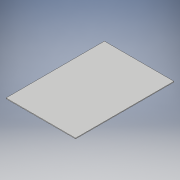
# Autodesk Inventor part: yaxis_platform_sheet
Saved by Autodesk Inventor 2019 (Build 230136000, 136)
## iProperties
Created: 2020-03-07
Part Number: yaxis_platform_sheet
Material: Generic
Document SubType Name: Modeling
Designer: nisha
Density: 1 g/cm^3
Appearance: Default
Author: nisha
Autodesk Inventor part; units mm, degrees
ref_plane "YZ Plane" through (0, 0, 0) normal (1, 0, 0) x (0, 1, 0)
ref_plane "XZ Plane" through (0, 0, 0) normal (0, 1, 0) x (-1, 0, 0)
ref_plane "XY Plane" through (0, 0, 0) normal (0, 0, 1) x (1, 0, 0)
sketch "Sketch1" plane through (0, 0, 0) normal (0, 1, 0) x (-1, 0, 0)
  line L0 (0, 0) -> (-210, 0)
  line L1 (-210, 0) -> (-210, -297)
  line L2 (-210, -297) -> (0, -297)
  line L3 (0, -297) -> (0, 0)
  dimension "d0" = 210
  dimension "d1" = 297
  dimension "d2" = 210
  dimension "d3" = 297
  constraints: 8 end point, 2 perpendicular, 1 horizontal
  measures "d0" distance of L0.start L0.end
  measures "d1" distance of L0.end L1.end
  measures "d2" distance of L1.end L2.end
  measures "d3" distance of L2.end L0.start
extrude "Extrusion1" add sketch "Sketch1" along normal blind 2
body "Solid1"
